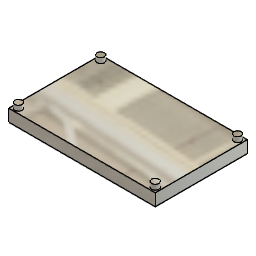
EcraVoldePrint (Autodesk Fusion 360 archive; units mm, degrees)
design "EcraVoldeprint"
Autodesk Fusion 360 part; units mm, degrees
sketch "Sketch1" plane through (0, 0, 0) normal (0, 1, 0) x (1, 0, 0)
  line L0 (60.5, -38) -> (-60.5, -38)
  line L1 (-60.5, -38) -> (-60.5, 38)
  line L2 (-60.5, 38) -> (60.5, 38)
  line L3 (60.5, 38) -> (60.5, -38)
  line L4 (60.5, -38) -> (-60.5, 38) construction
  line L5 (-60.5, -38) -> (60.5, 38) construction
  line L6 (56.5, -34) -> (-56.5, -34) construction
  line L7 (-56.5, -34) -> (-56.5, 34) construction
  line L8 (-56.5, 34) -> (56.5, 34) construction
  line L9 (56.5, 34) -> (56.5, -34) construction
  line L10 (56.5, -34) -> (-56.5, 34) construction
  line L11 (-56.5, -34) -> (56.5, 34) construction
  circle A0 centre (56.5, 34) radius 3
  circle A1 centre (56.5, -34) radius 3
  circle A2 centre (-56.5, -34) radius 3
  circle A3 centre (-56.5, 34) radius 3
  dimension "d1" = 121
  dimension "d2" = 76
  dimension "d3" = 113
  dimension "d4" = 68
  dimension "d5" = 6
  dimension "d6" = 6
  dimension "d7" = 6
  dimension "d8" = 6
  constraint horizontal L0
  constraint perpendicular L0 L1
  constraint parallel L0 L2
  constraint parallel L1 L3
  constraint coincident L4 origin
  constraint coincident L5 origin
  constraint horizontal L6
  constraint perpendicular L6 L7
  constraint parallel L6 L8
  constraint parallel L7 L9
  constraint coincident L10 origin
  constraint coincident L11 origin
  constraint coincident L8.end L9.start
  constraint coincident L6.start L9.end
  constraint coincident L6.end L7.start
  constraint coincident L7.end L8.start
  measures "d1" distance of L1.end L2.end
  measures "d2" distance of L0.end L1.end
  measures "d3" distance of L7.end L8.end
  measures "d4" distance of L6.end L7.end
  measures "d5" diameter of A0
  measures "d6" diameter of A1
  measures "d7" diameter of A2
  measures "d8" diameter of A3
extrude "Extrude1" add sketch "Sketch1" along normal blind 10
extrude "Extrude2" add sketch "Sketch1" along normal blind 14.2 contours A0 | A1 | A2 | A3
equation "d11 = 10 mm + 4.2 mm"
